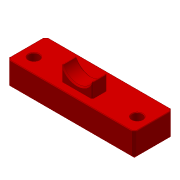
# Autodesk Inventor part: single extruder securer
Saved by Autodesk Inventor 2015 (Build 190159000, 159)
## iProperties
Created: 2020-04-10
Part Number: single extruder securer
Material: Generic
Document SubType Name: Modeling
Designer: Ghassan Yusuf
Density: 1 g/cm^3
Appearance: Default(1)
Author: Ghassan Yusuf
Autodesk Inventor part; units mm, degrees
ref_plane "YZ Plane" through (0, 0, 0) normal (1, 0, 0) x (0, 1, 0)
ref_plane "XZ Plane" through (0, 0, 0) normal (0, 1, 0) x (-1, 0, 0)
ref_plane "XY Plane" through (0, 0, 0) normal (0, 0, 1) x (1, 0, 0)
sketch "Sketch1" plane through (0, 0, 0) normal (0, 0, 1) x (1, 0, 0)
  line L0 (-24.65, 7.5) -> (24.65, 7.5)
  line L1 (24.65, 7.5) -> (24.65, -7.5)
  line L2 (24.65, -7.5) -> (-24.65, -7.5)
  line L3 (-24.65, -7.5) -> (-24.65, 7.5)
  circle A0 centre (-20, -1.7) radius 2
  circle A1 centre (20, -1.7) radius 2
  point P0 (0, 0)
  point P1 (-24.65, 0)
  point P2 (0, 7.5)
  dimension "d0" = 49.3
  dimension "d1" = 15
  dimension "d2" = 4
  dimension "d3" = 40
  dimension "d7" = 9.2
  dimension "d8" = 9.2
  dimension "d9" = 20
  constraints: 8 end point, 2 centre point, 2 horizontal alignment, 2 midpoint, 2 parallel, 1 equal radius, 1 horizontal, 1 perpendicular, 1 vertical alignment
  measures "d0" distance of L1.end L2.end
  measures "d1" distance of L0.end L1.end
  measures "d2" diameter of A0
  measures "d3" distance of A1.centre A0.centre
  measures "d7" distance from line of L0 A0.centre
  measures "d8" distance from line of A1.centre L0
  measures "d9" horizontal distance of point (0, 0) A0.centre
extrude "Extrusion1" add sketch "Sketch1" along normal mid plane 9.5
sketch "Sketch2" plane through (0, 0, 4.75) normal (0, 0, 1) x (1, 0, 0)
  line L0 (-6.65, 1.2) -> (5.65, 1.2)
  line L1 (5.65, 1.2) -> (5.65, -4.6)
  line L2 (5.65, -4.6) -> (-6.65, -4.6)
  line L3 (-6.65, -4.6) -> (-6.65, 1.2)
  line L4 (-24.65, 7.5) -> (24.65, 7.5) projected
  line L5 (24.65, -7.5) -> (24.65, 7.5) projected
  line L6 (-6.5, 1.2) -> (-6.5, -4.6)
  line L7 (-24.65, -7.5) -> (24.65, -7.5) projected
  line L8 (5.5, 1.2) -> (5.5, -4.6)
  point P0 (0, 0)
  dimension "d10" = 5.8
  dimension "d11" = 6.3
  dimension "d12" = 12.3
  dimension "d13" = 19
  dimension "d14" = 0.15
  constraints: 12 end point, 4 point on line, 2 parallel, 2 perpendicular, 1 horizontal, 1 vertical
  measures "d10" distance of L0.end L1.end
  measures "d11" distance between parallel lines of L4 L0
  measures "d12" distance between parallel lines of L1 L3
  measures "d13" distance between parallel lines of L5 L1
  measures "d14" distance between parallel lines of L3 L6
extrude "Extrusion3" add sketch "Sketch2" along normal blind 8 contours L0 L8 L2 L6
sketch "Sketch3" plane through (-6.5, 1.2, 4.75) normal (0, 1, 0) x (1, 0, 0)
  line L0 (0, -8) -> (12, -8) projected
  circle A0 centre (6, -8) radius 6.15
  point P0 (6.5, 4.75)
  dimension "d20" = 12.3
  constraints: 1 centre point, 1 midpoint
  measures "d20" diameter of A0
extrude "Extrusion4" cut sketch "Sketch3" against normal blind 8
chamfer "Chamfer1" distance 0.5 angle 45 4 edges at (-6.5, -4.6, 8.075) (-6.5, 1.2, 8.075) (5.5, 1.2, 8.075) (5.5, -4.6, 8.075)
chamfer "Chamfer2" distance 0.5 angle 45 2 edges at (-0.5, -4.6, 6.6) (-0.5, 1.2, 6.6)
fillet "Fillet1" radius 0.2 2 edges at (-6.5, -1.7, 11.4) (5.5, -1.7, 11.4)
chamfer "Chamfer3" distance 1 angle 45 8 edges at (24.65, 0, -4.75) (-24.65, 0, -4.75) (0, 7.5, -4.75) (24.65, 7.5, 0) (-24.65, 7.5, 0) (24.65, -7.5, 0) (0, -7.5, -4.75) (-24.65, -7.5, 0)
sketch "Sketch4" plane through (0, 0, -4.75) normal (0, 0, -1) x (-1, 0, 0)
  circle A0 centre (-20, -1.7) radius 2 projected
  circle A1 centre (-20, -1.7) radius 3
  circle A2 centre (20, -1.7) radius 2 projected
  circle A3 centre (20, -1.7) radius 3
  point P0 (0, 0)
  dimension "d33" = 6
  dimension "d34" = 6
  constraints: 2 centre point, 2 coincident
  measures "d33" diameter of A1
  measures "d34" diameter of A3
extrude "Extrusion5" cut sketch "Sketch4" against normal blind 3 contours A0 | A1 | A2 | A3
fillet "Fillet2" radius 0.2 8 edges at (0, 7.5, 4.75) (0, -7.5, 4.75) (-24.65, 0, 4.75) (24.65, 0, 4.75) (24.15, 7, 4.75) (24.15, -7, 4.75) (-24.15, -7, 4.75) (-24.15, 7, 4.75)
chamfer "Chamfer4" distance 0.2 angle 45 4 edges at (-22, -1.7, 4.75) (18, -1.7, 4.75) (-22, -1.7, -1.75) (18, -1.7, -1.75)
equation "\"d9\" = 0.5 * d3"
body "Solid1"
